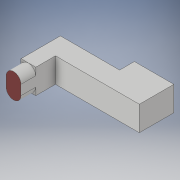
# Autodesk Inventor part: button_press
Saved by Autodesk Inventor 2017 (Build 210142000, 142)
## iProperties
Created: 2016-11-05
Part Number: button_press
Material: Generic
Document SubType Name: Modeling
Designer: radrajith
Density: 1 g/cm^3
Appearance: Default
Author: radrajith
Autodesk Inventor part; units mm, degrees
ref_plane "YZ Plane" through (0, 0, 0) normal (1, 0, 0) x (0, 1, 0)
ref_plane "XZ Plane" through (0, 0, 0) normal (0, 1, 0) x (-1, 0, 0)
ref_plane "XY Plane" through (0, 0, 0) normal (0, 0, 1) x (1, 0, 0)
sketch "Sketch1" plane through (0, 0, 0) normal (0, 0, 1) x (1, 0, 0)
  line L0 (0, 0) -> (20, 0)
  line L1 (20, 0) -> (20, 5)
  line L2 (20, 5) -> (0, 5)
  line L3 (0, 5) -> (0, 0)
  dimension "d0" = 20
  dimension "d1" = 5
  constraints: 8 end point, 2 parallel, 1 horizontal, 1 perpendicular
  measures "d0" distance of L2.end L1.end
  measures "d1" distance of L1.end L0.end
extrude "Extrusion1" add sketch "Sketch1" along normal blind 4
sketch "Sketch2" plane through (0, 0, 4) normal (0, 0, 1) x (1, 0, 0)
  line L0 (0, 0) -> (3, 0)
  line L1 (3, 0) -> (3, 5)
  line L2 (3, 5) -> (0, 5)
  line L3 (0, 5) -> (0, 0)
  dimension "d4" = 3
  dimension "d5" = 5
  constraints: 8 end point, 2 parallel, 1 horizontal, 1 perpendicular
  measures "d4" distance of L2.end L1.end
  measures "d5" distance of L1.end L0.end
extrude "Extrusion2" add sketch "Sketch2" along normal blind 4
sketch "Sketch3" plane through (0, 0, 8) normal (0, 0, 1) x (1, 0, 0)
  line L0 (1.5, 0) -> (1.5, 0)
  line L1 (3, 1.5) -> (3, 3.5)
  line L2 (1.5, 5) -> (1.5, 5)
  line L3 (0, 3.5) -> (0, 1.5)
  arc A0 (1.5, 5) -> (0, 3.5) centre (1.5, 3.5) ccw
  arc A1 (0, 1.5) -> (1.5, 0) centre (1.5, 1.5) ccw
  arc A2 (1.5, 0) -> (3, 1.5) centre (1.5, 1.5) ccw
  arc A3 (3, 3.5) -> (1.5, 5) centre (1.5, 3.5) ccw
  point P0 (0, 0)
  point P1 (3, 5)
  point P2 (3, 0)
  point P3 (0, 5)
  dimension "d8" = 3
  dimension "d9" = 5
  dimension "d10" = 1.5
  dimension "d11" = 1.5
  constraints: 8 end point, 8 point on circle, 8 point on line, 8 tangent, 4 centre point, 2 equal radius, 2 parallel, 1 horizontal, 1 perpendicular
  measures "d8" distance of point (0, 5) point (3, 5)
  measures "d9" distance of point (3, 5) point (3, 0)
  measures "d10" radius of A0
  measures "d11" radius of A1
extrude "Extrusion3" add sketch "Sketch3" along normal blind 3
sketch "Sketch5" plane through (0, 0, 0) normal (0, 0, -1) x (-1, 0, 0)
  line L0 (-20, 5) -> (-12, 5)
  line L1 (-12, 5) -> (-12, 0)
  line L2 (-12, 0) -> (-20, 0)
  line L3 (-20, 0) -> (-20, 5)
  point P0 (0, 0)
  constraints: 8 end point, 2 parallel, 1 horizontal, 1 perpendicular
extrude "Extrusion5" add sketch "Sketch5" along normal blind 3
body "Solid1"
